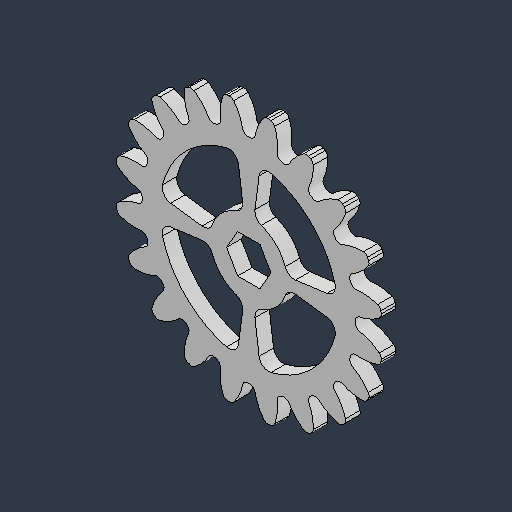
# Autodesk Inventor part: GEAR,DRIVE,INTAKE
Saved by Autodesk Inventor 2026 (Build 300175050, 175E)
## iProperties
Created: 2026-04-12
Part Number: GEAR,DRIVE,INTAKE
Material: Generic
Document SubType Name: Modeling
Designer: Jthib
Mass: 14.5016 g
Surface Area: 101.793 cm^2
Volume: 14.5016 cm^3
Density: 1 g/cm^3
Appearance: Default
Author: Jthib
Autodesk Inventor part; units mm, degrees
ref_plane "YZ Plane" through (0, 0, 0) normal (1, 0, 0) x (0, 1, 0)
ref_plane "XZ Plane" through (0, 0, 0) normal (0, 1, 0) x (-1, 0, 0)
ref_plane "XY Plane" through (0, 0, 0) normal (0, 0, 1) x (1, 0, 0)
sketch "Sketch1" plane through (0, 0, 0) normal (0, 0, 1) x (1, 0, 0)
  spline S0 degree 3 poles (-5.5615, 43.8176) (-5.4208, 43.6403) (-5.1393, 43.2859) (-4.7383, 42.738) (-4.3539, 42.1783) (-3.9895, 41.6053) (-3.6465, 41.0194) (-3.3273, 40.42) (-3.0351, 39.807) (-2.7742, 39.1801) (-2.5874, 38.6456) (-2.4633, 38.2104) (-2.3565, 37.7702) (-2.3075, 37.3192) (-2.2052, 36.8777) (-2.0974, 36.5554) (-1.9571, 36.2458) (-1.7812, 35.9543) (-1.5955, 35.7397) (-1.431, 35.5839) (-1.2942, 35.4832) (-1.1521, 35.3898) (-0.9983, 35.3173) (-0.8413, 35.2521) (-0.6762, 35.2116) (-0.5093, 35.1788) (-0.2827, 35.1697) (0, 35.1755) (0.2827, 35.1697) (0.5093, 35.1788) (0.6762, 35.2116) (0.8413, 35.2521) (0.9983, 35.3173) (1.1521, 35.3898) (1.2942, 35.4832) (1.431, 35.5839) (1.5955, 35.7397) (1.7812, 35.9543) (1.9571, 36.2458) (2.0974, 36.5554) (2.2052, 36.8777) (2.3075, 37.3192) (2.3565, 37.7702) (2.4633, 38.2104) (2.5874, 38.6456) (2.7742, 39.1801) (3.0351, 39.807) (3.3273, 40.42) (3.6465, 41.0194) (3.9895, 41.6053) (4.3539, 42.1783) (4.7383, 42.738) (5.1393, 43.2859) (5.4208, 43.6403) (5.5615, 43.8176) knots 0 0 0 0 0.067886 0.135771 0.203657 0.271542 0.339426 0.407309 0.475191 0.543071 0.610947 0.644889 0.678829 0.746701 0.780639 0.814577 0.848504 0.882427 0.916332 0.933308 0.950278 0.967249 0.984218 1.001186 1.018155 1.035124 1.052092 1.086035 1.119979 1.136946 1.153916 1.170884 1.187852 1.204822 1.221793 1.238763 1.255739 1.289644 1.323567 1.357493 1.391431 1.42537 1.493242 1.527182 1.561124 1.628999 1.696879 1.764761 1.832645 1.900529 1.968414 2.036299 2.104185 2.172071 2.172071 2.172071 2.172071
  circle A0 centre (0, 0) radius 35.1732 construction
  circle A1 centre (0, 0) radius 37.5877 construction
  circle A2 centre (0, 0) radius 40 construction
  circle A3 centre (0, 0) radius 44.1691
  point P0 (-5.1429, 43.2832)
  point P1 (-4.7411, 42.736)
  point P2 (-4.3573, 42.1761)
  point P3 (-3.9931, 41.6032)
  point P4 (-3.6505, 41.0171)
  point P5 (-3.3318, 40.4177)
  point P6 (-3.0403, 39.8047)
  point P7 (-2.7803, 39.1776)
  point P8 (-2.5585, 38.5361)
  point P9 (-2.4655, 38.2097)
  point P10 (-2.388, 37.8793)
  point P11 (-2.2775, 37.2096)
  point P12 (-2.2, 36.8792)
  point P13 (-2.092, 36.5575)
  point P14 (-1.9512, 36.2488)
  point P15 (-1.7734, 35.9599)
  point P16 (-1.5531, 35.7022)
  point P17 (-1.4287, 35.5866)
  point P18 (-1.2933, 35.4844)
  point P19 (-1.1501, 35.3933)
  point P20 (-0.9978, 35.3185)
  point P21 (-0.8399, 35.2562)
  point P22 (-0.6759, 35.2129)
  point P23 (-0.5088, 35.1831)
  point P24 (-0.3394, 35.1731)
  point P25 (0, 35.1732)
  point P26 (0.3394, 35.1731)
  point P27 (0.5088, 35.1831)
  point P28 (0.6759, 35.2129)
  point P29 (0.8399, 35.2562)
  point P30 (0.9978, 35.3185)
  point P31 (1.1501, 35.3933)
  point P32 (1.2933, 35.4844)
  point P33 (1.4287, 35.5866)
  point P34 (1.5531, 35.7022)
  point P35 (1.7734, 35.9599)
  point P36 (1.9512, 36.2488)
  point P37 (2.092, 36.5575)
  point P38 (2.2, 36.8792)
  point P39 (2.2775, 37.2096)
  point P40 (2.388, 37.8793)
  point P41 (2.4655, 38.2097)
  point P42 (2.5585, 38.5361)
  point P43 (2.7803, 39.1776)
  point P44 (3.0403, 39.8047)
  point P45 (3.3318, 40.4177)
  point P46 (3.6505, 41.0171)
  point P47 (3.9931, 41.6032)
  point P48 (4.3573, 42.1761)
  point P49 (4.7411, 42.736)
  point P50 (5.1429, 43.2832)
  constraints: 4 centre point, 2 point on circle, 111 other
extrude "Extrusion1" add sketch "Sketch1" against normal blind 4.7625
extrude "Extrusion2" cut sketch "Sketch1" along normal through all both and the other way through all contours A3 S0 picked at (-0.9019, 41.2981)
fillet "Fillet1" radius 1.5875 2 edges at (-5.5615, 43.8176, -2.3813) (5.5615, 43.8176, -2.3813)
pattern_circular "Circular Pattern1" count 20 over 360 about axis through (0, 0, -10) along (0, 0, 1) of "Extrusion2", "Fillet1"
sketch "Sketch3" plane through (0, 0, 0) normal (0, 0, 1) x (1, 0, 0)
  line L0 (3.6662, 6.35) -> (7.3323, 0)
  line L1 (7.3323, 0) -> (3.6662, -6.35)
  line L2 (3.6662, -6.35) -> (-3.6662, -6.35)
  line L3 (-3.6662, -6.35) -> (-7.3323, 0)
  line L4 (-7.3323, 0) -> (-3.6662, 6.35)
  line L5 (-3.6662, 6.35) -> (3.6662, 6.35)
  point P0 (0, 0)
  point P1 (0, 0)
  dimension "d9" = 12.7
  constraints: 12 end point, 1 coincident, 1 horizontal, 13 other
  measures "d9" distance between parallel lines of L2 L5
extrude "Extrusion3" cut sketch "Sketch3" against normal through all
sketch "Sketch4" plane through (0, 0, -4.7625) normal (0, 0, -1) x (-1, 0, 0)
  circle A0 centre (0, 0) radius 12.7
  circle A1 centre (0, 0) radius 29.3687
  line L0 (-12.5913, 1.6577) -> (-29.1175, 3.8334)
  line L1 (-1.6577, 12.5913) -> (-3.8334, 29.1175)
  line L2 (0, -88.9) -> (0, 88.9) construction
  line L3 (-88.9, 0) -> (88.9, 0) construction
  point P0 (-3.287, 12.2673)
  point P1 (-12.2673, 3.287)
  dimension "d13" = 7.5
  dimension "d14" = 7.5
  dimension "d15" = 75
  dimension "d16" = 58.7375
  dimension "d17" = 25.4
  dimension "d7" = 127
  constraints: 4 end point, 4 point on circle, 2 centre point, 2 coincident, 2 line through centre
  measures "d13" angle of L0 L3
  measures "d14" angle of L2 L1
  measures "d15" angle of L1 L0
  measures "d16" diameter of A1
  measures "d17" diameter of A0
extrude "Extrusion4" cut sketch "Sketch4" against normal blind 25.4 contours A0 L0 A1 L1 picked at (-23.1021, 5.1786)
fillet "Fillet2" radius 3.175 4 edges at (29.1175, 3.8334, -2.3813) (3.8334, 29.1175, -2.3813) (12.5913, 1.6577, -2.3813) (1.6577, 12.5913, -2.3813)
pattern_circular "Circular Pattern2" count 4 over 360 about axis through (0, 0, -10) along (0, 0, 1) of "Extrusion4", "Fillet2"
equation "\"d0\" = FaceWidth"
equation "\"d13\" = d14"
equation "\"d7\" = PitchDiameter"
equation "\"Module\" = 4"
equation "\"PressureAngle\" = 20deg"
equation "\"UnitProfileClearance\" = 0.25"
equation "\"UnitRoundRadius\" = 0.35"
equation "\"HeadDiameter\" = 88.33821"
equation "\"RootDiameter\" = 70.34632"
equation "\"BaseDiameter\" = 75.17541"
equation "\"PitchDiameter\" = 127"
equation "\"FaceWidth\" = 4.7625"
equation "\"HelixAngle\" = 0"
equation "\"UnitCorrection\" = 0.043289"
equation "\"UnitAddendumModification\" = 0.001013"
equation "\"CircularPitch\" = 12.56637"
equation "\"UnitBacklashShift\" = 0"
equation "\"TotalToolShift\" = 0.17316"
equation "\"IsInternal\" = 0"
body "Solid1"
